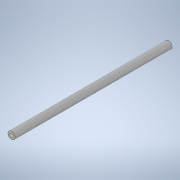
# Autodesk Inventor part: Main Screw
Saved by Autodesk Inventor 2021 (Build 250183000, 183)
## iProperties
Created: 2021-02-01
Part Number: Main Screw
Material: Generic
Document SubType Name: Modeling
Designer: chris
Density: 1 g/cm^3
Appearance: Default
Author: chris
Autodesk Inventor part; units mm, degrees
ref_plane "YZ Plane" through (0, 0, 0) normal (1, 0, 0) x (0, 1, 0)
ref_plane "XZ Plane" through (0, 0, 0) normal (0, 1, 0) x (-1, 0, 0)
ref_plane "XY Plane" through (0, 0, 0) normal (0, 0, 1) x (1, 0, 0)
sketch "Sketch1" plane through (0, 0, 0) normal (0, 0, 1) x (1, 0, 0)
  circle A0 centre (0, 0) radius 5
  circle A1 centre (0, 0) radius 2.5
  dimension "d0" = 10
  dimension "d1" = 5
  constraints: 2 centre point, 2 coincident
  measures "d0" diameter of A0
  measures "d1" diameter of A1
extrude "Extrusion1" add sketch "Sketch1" along normal blind 215
thread "Thread1" size "M10x1.5" class "6g" standard "ANSI Metric M Profile" full length
sketch "Sketch2" plane through (0, 0, 215) normal (0, 0, 1) x (1, 0, 0)
  point P0 (0, 0)
sketch "Sketch3" plane through (0, 0, 0) normal (0, 0, -1) x (-1, 0, 0)
  circle A0 centre (0, 0) radius 2.5 projected
  line L0 (-2.2913, 1) -> (2.2913, 1)
  arc A1 (2.2913, 1) -> (-2.2913, 1) centre (0, 0) ccw
  dimension "d6" = 1
  constraints: 4 point on circle, 2 end point, 1 centre point, 1 concentric, 1 horizontal
  measures "d6" distance from line of A0.centre L0
extrude "Extrusion2" add sketch "Sketch3" against normal blind 15 contours L0 A0 picked at (0.6667, 1.1666)
body "Solid1"
